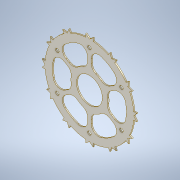
# Autodesk Inventor part: Wood Magnets  (UNI) V1.0.
Saved by Autodesk Inventor 2022.1 (Build 261234020, 234B)
## iProperties
Created: 2022-03-16
Part Number: Wood Magnets  (UNI) V1.0.
Material: Titanium
Document SubType Name: Modeling
Designer: NCai2
Density: 4.51 g/cm^3
Appearance: Titanium
Mass: 5.57938 g
Surface Area: 30.6065 cm^2
Volume: 1.23711 cm^3
Author: NCai2
Autodesk Inventor part; units mm, degrees
ref_plane "YZ Plane" through (0, 0, 0) normal (1, 0, 0) x (0, 1, 0)
ref_plane "XZ Plane" through (0, 0, 0) normal (0, 1, 0) x (-1, 0, 0)
ref_plane "XY Plane" through (0, 0, 0) normal (0, 0, 1) x (1, 0, 0)
sketch "Sketch1" plane through (0, 0, 0) normal (0, 0, 1) x (1, 0, 0)
  circle A0 centre (0, 0) radius 38.1
  circle A1 centre (0, 0) radius 31.75
  circle A2 centre (0, 0) radius 15.875
  line L0 (0, 0) -> (0, 38.1) construction
  circle A3 centre (0, 31.75) radius 1.5
  line L1 (-1.5875, 15.7954) -> (-1.5875, 38.0669)
  line L2 (1.5875, 15.7954) -> (1.5875, 38.0669)
  arc A4 (9.9219, 30.1599) -> (1.5875, 24.1279) centre (7.9375, 24.1279) ccw
  arc A5 (-1.5875, 24.1279) -> (-9.9219, 30.1599) centre (-7.9375, 24.1279) ccw
  arc A6 (1.5875, 20.7593) -> (5.6696, 14.828) centre (7.9375, 20.7593) ccw
  arc A7 (-5.6696, 14.828) -> (-1.5875, 20.7593) centre (-7.9375, 20.7593) ccw
  circle A8 centre (0, 0) radius 11.1125
  line L3 (-1.5875, 38.0669) -> (-1.5875, 40.6069) construction
  line L4 (-1.5875, 40.6069) -> (1.5875, 38.0669) construction
  line L5 (0, 38.1) -> (-3.175, 38.1) construction
  line L6 (-3.175, 38.1) -> (-3.175, 40.6069) construction
  line L7 (-3.175, 40.6069) -> (0, 40.6069) construction
  line L8 (0, 40.6069) -> (0, 38.1) construction
  line L9 (0, 38.1) -> (-3.175, 40.6069)
  line L10 (-3.175, 37.9675) -> (-3.175, 40.6069)
  line L11 (0, 38.1) -> (3.175, 40.6069)
  line L12 (3.175, 37.9675) -> (3.175, 40.6069)
  line L13 (-19.05, 32.9956) -> (-17.5538, 36.7541)
  line L14 (-16.2341, 34.4683) -> (-17.5538, 36.7541)
  line L15 (-19.05, 32.9956) -> (-23.0531, 33.5791)
  line L16 (-21.7334, 31.2933) -> (-23.0531, 33.5791)
  line L17 (-32.9956, 19.05) -> (-33.5791, 23.0531)
  line L18 (-31.2933, 21.7334) -> (-33.5791, 23.0531)
  line L19 (-32.9956, 19.05) -> (-36.7541, 17.5538)
  line L20 (-34.4683, 16.2341) -> (-36.7541, 17.5538)
  line L21 (-38.1, 0) -> (-40.6069, 3.175)
  line L22 (-37.9675, 3.175) -> (-40.6069, 3.175)
  line L23 (-38.1, 0) -> (-40.6069, -3.175)
  line L24 (-37.9675, -3.175) -> (-40.6069, -3.175)
  line L25 (-32.9956, -19.05) -> (-36.7541, -17.5538)
  line L26 (-34.4683, -16.2341) -> (-36.7541, -17.5538)
  line L27 (-32.9956, -19.05) -> (-33.5791, -23.0531)
  line L28 (-31.2933, -21.7334) -> (-33.5791, -23.0531)
  line L29 (-19.05, -32.9956) -> (-23.0531, -33.5791)
  line L30 (-21.7334, -31.2933) -> (-23.0531, -33.5791)
  line L31 (-19.05, -32.9956) -> (-17.5538, -36.7541)
  line L32 (-16.2341, -34.4683) -> (-17.5538, -36.7541)
  line L33 (0, -38.1) -> (-3.175, -40.6069)
  line L34 (-3.175, -37.9675) -> (-3.175, -40.6069)
  line L35 (0, -38.1) -> (3.175, -40.6069)
  line L36 (3.175, -37.9675) -> (3.175, -40.6069)
  line L37 (19.05, -32.9956) -> (17.5538, -36.7541)
  line L38 (16.2341, -34.4683) -> (17.5538, -36.7541)
  line L39 (19.05, -32.9956) -> (23.0531, -33.5791)
  line L40 (21.7334, -31.2933) -> (23.0531, -33.5791)
  line L41 (32.9956, -19.05) -> (33.5791, -23.0531)
  line L42 (31.2933, -21.7334) -> (33.5791, -23.0531)
  line L43 (32.9956, -19.05) -> (36.7541, -17.5538)
  line L44 (34.4683, -16.2341) -> (36.7541, -17.5538)
  line L45 (38.1, 0) -> (40.6069, -3.175)
  line L46 (37.9675, -3.175) -> (40.6069, -3.175)
  line L47 (38.1, 0) -> (40.6069, 3.175)
  line L48 (37.9675, 3.175) -> (40.6069, 3.175)
  line L49 (32.9956, 19.05) -> (36.7541, 17.5538)
  line L50 (34.4683, 16.2341) -> (36.7541, 17.5538)
  line L51 (32.9956, 19.05) -> (33.5791, 23.0531)
  line L52 (31.2933, 21.7334) -> (33.5791, 23.0531)
  line L53 (19.05, 32.9956) -> (23.0531, 33.5791)
  line L54 (21.7334, 31.2933) -> (23.0531, 33.5791)
  line L55 (19.05, 32.9956) -> (17.5538, 36.7541)
  line L56 (16.2341, 34.4683) -> (17.5538, 36.7541)
  arc A9 (-21.1583, 23.6725) -> (-20.1016, 13.4388) centre (-16.9266, 18.938) ccw
  line L57 (-12.8855, 9.2725) -> (-32.1732, 20.4083)
  line L58 (-14.473, 6.5229) -> (-33.7607, 17.6586)
  circle A10 centre (-27.4963, 15.875) radius 1.5
  arc A11 (-21.6891, 10.6891) -> (-31.0802, 6.4873) centre (-24.8641, 5.1899) ccw
  arc A12 (-15.6763, 2.504) -> (-18.7718, 9.0048) centre (-21.9468, 3.5056) ccw
  arc A13 (-17.1843, 11.7544) -> (-10.0066, 12.3241) centre (-14.0093, 17.2537) ccw
  arc A14 (-31.0802, -6.4873) -> (-21.6891, -10.6891) centre (-24.8641, -5.1899) ccw
  line L59 (-14.473, -6.5229) -> (-33.7607, -17.6586)
  line L60 (-12.8855, -9.2725) -> (-32.1732, -20.4083)
  circle A15 centre (-27.4963, -15.875) radius 1.5
  arc A16 (-20.1016, -13.4388) -> (-21.1583, -23.6725) centre (-16.9266, -18.938) ccw
  arc A17 (-10.0066, -12.3241) -> (-17.1843, -11.7544) centre (-14.0093, -17.2537) ccw
  arc A18 (-18.7718, -9.0048) -> (-15.6763, -2.504) centre (-21.9468, -3.5056) ccw
  arc A19 (-9.9219, -30.1599) -> (-1.5875, -24.1279) centre (-7.9375, -24.1279) ccw
  line L61 (-1.5875, -15.7954) -> (-1.5875, -38.0669)
  line L62 (1.5875, -15.7954) -> (1.5875, -38.0669)
  circle A20 centre (0, -31.75) radius 1.5
  arc A21 (1.5875, -24.1279) -> (9.9219, -30.1599) centre (7.9375, -24.1279) ccw
  arc A22 (5.6696, -14.828) -> (1.5875, -20.7593) centre (7.9375, -20.7593) ccw
  arc A23 (-1.5875, -20.7593) -> (-5.6696, -14.828) centre (-7.9375, -20.7593) ccw
  arc A24 (21.1583, -23.6725) -> (20.1016, -13.4388) centre (16.9266, -18.938) ccw
  line L63 (12.8855, -9.2725) -> (32.1732, -20.4083)
  line L64 (14.473, -6.5229) -> (33.7607, -17.6586)
  circle A25 centre (27.4963, -15.875) radius 1.5
  arc A26 (21.6891, -10.6891) -> (31.0802, -6.4873) centre (24.8641, -5.1899) ccw
  arc A27 (15.6763, -2.504) -> (18.7718, -9.0048) centre (21.9468, -3.5056) ccw
  arc A28 (17.1843, -11.7544) -> (10.0066, -12.3241) centre (14.0093, -17.2537) ccw
  arc A29 (31.0802, 6.4873) -> (21.6891, 10.6891) centre (24.8641, 5.1899) ccw
  line L65 (14.473, 6.5229) -> (33.7607, 17.6586)
  line L66 (12.8855, 9.2725) -> (32.1732, 20.4083)
  circle A30 centre (27.4963, 15.875) radius 1.5
  arc A31 (20.1016, 13.4388) -> (21.1583, 23.6725) centre (16.9266, 18.938) ccw
  arc A32 (10.0066, 12.3241) -> (17.1843, 11.7544) centre (14.0093, 17.2537) ccw
  arc A33 (18.7718, 9.0048) -> (15.6763, 2.504) centre (21.9468, 3.5056) ccw
  point P0 (-27.9529, 15.0565)
  point P1 (-5.6696, 14.828)
  point P2 (0, 0)
  point P3 (-21.7334, 31.2933)
  point P4 (-19.05, 32.9956)
  point P5 (-34.4683, 16.2341)
  point P6 (-32.9956, 19.05)
  point P7 (-32.9956, 19.05)
  point P8 (-37.9675, -3.175)
  point P9 (-38.1, 0)
  point P10 (-38.1, 0)
  point P11 (-37.9675, 3.175)
  point P12 (-31.2933, -21.7334)
  point P13 (-32.9956, -19.05)
  point P14 (-16.2341, -34.4683)
  point P15 (-19.05, -32.9956)
  point P16 (-19.05, -32.9956)
  point P17 (-21.7334, -31.2933)
  point P18 (3.175, -37.9675)
  point P19 (0, -38.1)
  point P20 (0, -38.1)
  point P21 (-3.175, -37.9675)
  point P22 (21.7334, -31.2933)
  point P23 (19.05, -32.9956)
  point P24 (16.2341, -34.4683)
  point P25 (32.9956, -19.05)
  point P26 (32.9956, -19.05)
  point P27 (31.2933, -21.7334)
  point P28 (38.1, 0)
  point P29 (38.1, 0)
  point P30 (37.9675, 3.175)
  point P31 (31.2933, 21.7334)
  point P32 (32.9956, 19.05)
  point P33 (32.9956, 19.05)
  point P34 (34.4683, 16.2341)
  point P35 (19.05, 32.9956)
  point P36 (21.7334, 31.2933)
  point P37 (3.175, 37.9675)
  point P38 (-10.0066, 12.3241)
  point P39 (-21.1583, 23.6725)
  point P40 (-9.9219, 30.1599)
  point P41 (1.5875, -24.1279)
  point P42 (1.5875, -20.7593)
  point P43 (5.6696, -14.828)
  point P44 (9.9219, -30.1599)
  point P45 (15.6763, 2.504)
  point P46 (31.0802, -6.4873)
  point P47 (-20.1016, -13.4388)
  point P48 (-10.0066, -12.3241)
  point P49 (-5.6696, -14.828)
  point P50 (-21.1583, -23.6725)
  point P51 (-21.6891, 10.6891)
  point P52 (-18.7718, 9.0048)
  point P53 (-15.6763, 2.504)
  point P54 (-15.6763, -2.504)
  point P55 (10.0066, 12.3241)
  dimension "d0" = 76.2
  dimension "d1" = 63.5
  dimension "d2" = 31.75
  dimension "d3" = 3
  dimension "d4" = 1.5875
  dimension "d5" = 1.5875
  dimension "d10" = 22.225
  dimension "d15" = 2.54
  dimension "d22" = 3.175
  dimension "d25" = 360
  dimension "d27" = 6.35
  dimension "d28" = 6.35
  dimension "d31" = 360
  constraints: 134 end point, 54 point on circle, 33 centre point, 14 point on line, 8 symmetric about line, 4 parallel, 4 tangent, 3 coincident, 2 perpendicular, 2 vertical, 1 horizontal, 1 midpoint, 262 other
  measures "d1" diameter of A1
  measures "d2" diameter of A2
  measures "d3" diameter of A3
  measures "d4" distance between parallel lines of L0 L1
  measures "d5" distance between parallel lines of L0 L2
  measures "d10" diameter of A8
  measures "d15" distance of L1.end L3.end
  measures "d22" distance of L6.end L7.end
  measures "d27" radius of A6
  measures "d28" radius of A4
extrude "Extrusion1" add sketch "Sketch1" along normal blind 1 contours A0 L64 A1 L65 | L45 L46 A0 | A0 L48 L47 | A0 L49 L50 | L44 L43 A0 | L65 A1 A30 L66 A0 | A0 L63 A1 A25 L64 | A0 L52 L51 | L65 A2 L66 A1 A30 | A1 A29 L65 | L41 L42 A0 | L64 A26 A1 | A1 A25 L63 A2 L64 | L66 A1 L2 A0 | A0 L62 A1 L63 | L66 A31 A1 | A33 A2 L65 | A1 A24 L63 | L64 A2 A27 | A0 L53 L54 | A2 | L40 L39 A0 | A0 L56 L55 | A4 L2 A1 | L66 A2 A32 | L37 L38 A0 | A1 L62 A21 | A28 A2 L63 | L2 A2 L1 A1 A3 | A1 A3 L1 A0 L2 | L62 A0 L61 A1 A20 | A1 A20 L61 A2 L62 | A0 L11 L12 | A6 A2 L2 | L36 L35 A0 | L62 A2 A22 | A0 L10 L9 | L33 L34 A0 | L1 A5 A1 | A1 L57 A0 L1 | A2 A7 L1 | L61 A0 L60 A1 | A1 A19 L61 | L61 A23 A2 | A9 L57 A1 | A0 L13 L14 | A2 L57 A13 | A1 L60 A16 | L32 L31 A0 | A17 L60 A2 | L57 A2 L58 A1 A10 | A1 A10 L58 A0 L57 | A0 L16 L15 | L60 A0 L59 A1 A15 | A1 A15 L59 A2 L60 | L29 L30 A0 | A0 L17 L18 | A2 A12 L58 | A0 L28 L27 | L59 A18 A2 | A0 L20 L19 | L25 L26 A0 | L58 A11 A1 | A1 L59 A0 L58 | A1 A14 L59 | A0 L21 L22 | L24 L23 A0
body "Solid1"
